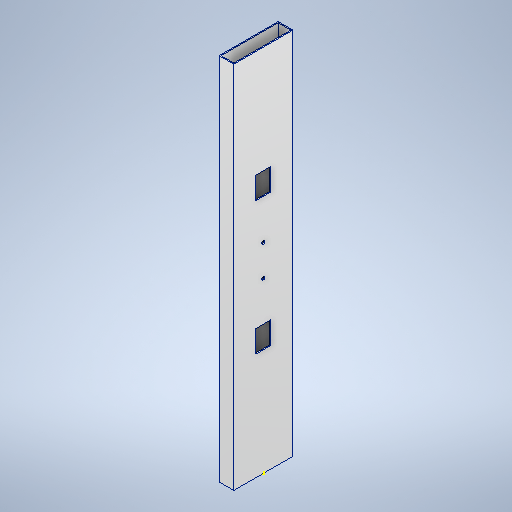
# Autodesk Inventor part: belka
Saved by Autodesk Inventor 2025 (Build 290162000, 162)
## iProperties
Created: 2024-04-16
Part Number: belka
Material: Aluminium 6061
Document SubType Name: Modeling
Designer: user
Density: 2.7 g/cm^3
Appearance: Aluminium — płaski
Author: user
Autodesk Inventor part; units mm, degrees
ref_plane "YZ Plane" through (0, 0, 0) normal (1, 0, 0) x (0, 1, 0)
ref_plane "XZ Plane" through (0, 0, 0) normal (0, 1, 0) x (-1, 0, 0)
ref_plane "XY Plane" through (0, 0, 0) normal (0, 0, 1) x (1, 0, 0)
sketch "Szkic2" plane through (0, 0, 0) normal (0, 1, 0) x (-1, 0, 0)
  line L0 (10, 40) -> (-10, 40)
  line L1 (-10, 40) -> (-10, -40)
  line L2 (-10, -40) -> (10, -40)
  line L3 (10, -40) -> (10, 40)
  line L4 (10, 40) -> (-10, -40) construction
  line L5 (-10, 40) -> (10, -40) construction
  line L6 (8.6, 38.6) -> (-8.6, 38.6)
  line L7 (-8.6, 38.6) -> (-8.6, -38.6)
  line L8 (-8.6, -38.6) -> (8.6, -38.6)
  line L9 (8.6, -38.6) -> (8.6, 38.6)
  line L10 (8.6, 38.6) -> (-8.6, -38.6) construction
  line L11 (-8.6, 38.6) -> (8.6, -38.6) construction
  point P0 (0, 0)
  point P1 (0, -40)
  dimension "d14" = 20
  dimension "d15" = 80
  dimension "d16" = 1.4
  dimension "d17" = 1.4
  constraints: 24 end point, 5 midpoint, 4 parallel, 2 horizontal, 2 perpendicular
  measures "d14" distance of L2.end L1.end
  measures "d15" distance of L1.end L0.end
  measures "d16" distance from line of point (0, -40) L8
  measures "d17" distance between parallel lines of L3 L9
extrude "Wyciągnięcie proste2" add sketch "Szkic2" along normal blind 500
sketch "Szkic3" plane through (-10, 0, -40) normal (-1, 0, 0) x (0, 0, 1)
  circle A0 centre (40, 229) radius 2.25
  circle A1 centre (40, 271) radius 2.25
  line L0 (0, 0) -> (0, 500) projected
  line L1 (0, 500) -> (80, 500) projected
  point P0 (40, 0)
  point P1 (40, 250)
  point P2 (40, 500)
  dimension "d20" = 4.5
  dimension "d21" = 4.5
  dimension "d22" = 21
  dimension "d23" = 21
  dimension "d24" = 40
  dimension "d25" = 40
  dimension "d26" = 40
  dimension "d27" = 250
  constraints: 2 centre point, 1 midpoint
  measures "d20" diameter of A0
  measures "d21" diameter of A1
  measures "d22" distance of point (40, 250) A0.centre
  measures "d23" distance of A1.centre point (40, 250)
  measures "d24" distance from line of L0 A0.centre
  measures "d25" distance from line of L0 A1.centre
  measures "d26" distance from line of L0 point (40, 250)
  measures "d27" distance of point (40, 500) point (40, 250)
extrude "Wyciągnięcie proste3" cut sketch "Szkic3" against normal blind 20
sketch "Szkic4" plane through (-10, 0, -40) normal (-1, 0, 0) x (0, 0, 1)
  point P0 (40, 0)
sketch "Szkic5" plane through (10, 0, 40) normal (1, 0, 0) x (0, 0, -1)
  point P0 (40, 0)
sketch "Szkic6" plane through (10, 0, 40) normal (1, 0, 0) x (0, 0, -1)
  point P0 (40, 0)
sketch "Szkic7" plane through (10, 0, 40) normal (1, 0, 0) x (0, 0, -1)
  line L0 (80, 0) -> (80, 500) projected
  line L1 (80, 250) -> (0, 250)
  line L2 (1.4, 0) -> (1.4, 500) projected
  line L3 (80, 250) -> (160, 250) construction
  line L4 (50, 355) -> (30, 355)
  line L5 (30, 355) -> (30, 325)
  line L6 (30, 325) -> (50, 325)
  line L7 (50, 325) -> (50, 355)
  line L8 (50, 355) -> (30, 325) construction
  line L9 (30, 355) -> (50, 325) construction
  line L10 (50, 145) -> (30, 145)
  line L11 (30, 145) -> (30, 175)
  line L12 (30, 175) -> (50, 175)
  line L13 (50, 175) -> (50, 145)
  point P0 (40, 0)
  point P1 (40, 340)
  dimension "d30" = 80
  dimension "d31" = 180
  dimension "d32" = 20
  dimension "d33" = 30
  dimension "d34" = 90
  dimension "d35" = 40
  constraints: 24 end point, 4 symmetric about line, 3 midpoint, 2 horizontal, 2 parallel, 2 perpendicular, 1 collinear
  measures "d30" distance of L1.start L1.end
  measures "d31" angle of L1 L3
  measures "d32" distance of L6.end L5.end
  measures "d33" distance of L5.end L4.end
  measures "d34" distance from line of L1 point (40, 340)
  measures "d35" distance from line of L0 point (40, 340)
extrude "Wyciągnięcie proste4" cut sketch "Szkic7" against normal blind 1.4
sketch "Szkic8" plane through (-10, 0, -40) normal (-1, 0, 0) x (0, 0, 1)
  line L0 (0, 0) -> (0, 500) projected
  line L1 (0, 250) -> (80, 250)
  line L2 (80, 0) -> (80, 500) projected
  line L3 (0, 250) -> (80, 250) construction
  circle A0 centre (40, 40) radius 10
  line L4 (0, 0) -> (80, 0) projected
  circle A1 centre (40, 460) radius 10
  point P0 (40, 0)
  point P1 (40, 0)
  dimension "d38" = 80
  dimension "d39" = 0
  dimension "d40" = 20
  dimension "d41" = 40
  dimension "d42" = 40
  constraints: 4 end point, 2 centre point, 2 midpoint, 1 collinear, 1 horizontal, 1 perpendicular, 1 symmetric about line, 1 other
  measures "d38" distance of L1.start L1.end
  measures "d39" distance between parallel lines of L1 L3
  measures "d40" diameter of A0
  measures "d41" distance of point (40, 0) A0.centre
  measures "d42" distance from line of L2 A0.centre
extrude "Wyciągnięcie proste5" cut sketch "Szkic8" against normal blind 1.4 contours A0 | A1
